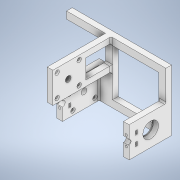
# Autodesk Inventor part: WinderBase
Saved by Autodesk Inventor 2021 (Build 250183000, 183)
## iProperties
Created: 2021-03-09
Part Number: WinderBase
Material: Generic
Document SubType Name: Modeling
Designer: elmar
Density: 1 g/cm^3
Appearance: White
Author: elmar
Autodesk Inventor part; units mm, degrees
ref_plane "YZ Plane" through (0, 0, 0) normal (1, 0, 0) x (0, 1, 0)
ref_plane "XZ Plane" through (0, 0, 0) normal (0, 1, 0) x (-1, 0, 0)
ref_plane "XY Plane" through (0, 0, 0) normal (0, 0, 1) x (1, 0, 0)
sketch "Sketch1" plane through (0, 0, 0) normal (0, 0, 1) x (1, 0, 0)
  line L0 (51, -43) -> (-51, -43)
  line L1 (-51, -43) -> (-51, 43)
  line L2 (-51, 43) -> (51, 43)
  line L3 (51, 43) -> (51, -43)
  line L4 (51, -43) -> (-51, 43) construction
  line L5 (-51, -43) -> (51, 43) construction
  point P0 (0, 0)
  dimension "d2" = 102
  dimension "d3" = 86
  constraints: 12 end point, 2 midpoint, 2 parallel, 1 horizontal, 1 perpendicular
  measures "d2" distance of L1.end L2.end
  measures "d3" distance of L0.end L1.end
extrude "Extrusion1" add sketch "Sketch1" along normal blind 8
sketch "Sketch4" plane through (0, 0, 8) normal (0, 0, 1) x (1, 0, 0)
  line L0 (-34.25, 43) -> (-26.25, 43)
  line L1 (-26.25, 43) -> (-26.25, 0)
  line L2 (-26.25, 0) -> (-34.25, 0)
  line L3 (-34.25, 0) -> (-34.25, 43)
  line L4 (51, 43) -> (-51, 43) projected
  line L5 (-51, 43) -> (-51, -43) projected
  point P0 (0, 0)
  dimension "d22" = 8
  dimension "d23" = 43
  dimension "d135" = 34.25
  constraints: 8 end point, 2 parallel, 1 collinear, 1 horizontal, 1 perpendicular
  measures "d22" distance of L0.start L0.end
  measures "d23" distance of L2.end L0.start
  measures "d135" distance from line of L3 point (0, 0)
extrude "Extrusion3" add sketch "Sketch4" along normal blind 82
sketch "Sketch5" plane through (-26.25, 0, 8) normal (1, 0, 0) x (0, 0, -1)
  circle A0 centre (-60.5, 21.5) radius 21.5
  line L0 (0, 43) -> (-82, 43) projected
  line L1 (-82, 0) -> (-82, 43) projected
  line L2 (0, 0) -> (-82, 0) projected
  line L3 (-45, 6) -> (-76, 6)
  line L4 (-76, 6) -> (-76, 37)
  line L5 (-76, 37) -> (-45, 37)
  line L6 (-45, 37) -> (-45, 6)
  line L7 (-45, 6) -> (-76, 37) construction
  line L8 (-76, 6) -> (-45, 37) construction
  point P0 (8, 0)
  dimension "d26" = 31
  constraints: 12 end point, 3 tangent, 2 midpoint, 2 parallel, 2 perpendicular, 1 centre point, 1 horizontal
  measures "d26" distance of L4.end L5.end
hole "Hole2" at (-26.25, 37, 84) at (-26.25, 37, 53) at (-26.25, 6, 53) at (-26.25, 6, 84) direction (-1, 0, 0) diameter 3.2 end through all countersink diameter 6.3 countersink angle 90 clearance for "Flat Head Machine Screw" size "M3" standard "Ansi Metric M Profile"
sketch "Sketch6" plane through (-34.25, 0, 8) normal (-1, 0, 0) x (0, 0, 1)
  point P0 (-8, 0)
  point P1 (60.5, 21.5)
hole "Hole3" at (-34.25, 21.5, 68.5) direction (1, 0, 0) diameter 8 end through all counterbore diameter 23 counterbore depth 2.2
sketch "Sketch8" plane through (0, 0, 8) normal (0, 0, 1) x (1, 0, 0)
  line L0 (51, -43) -> (51, 43) projected
  line L1 (51, -43) -> (43, -43)
  line L2 (43, -43) -> (43, 0)
  line L3 (43, 0) -> (51, 0)
  line L4 (51, 0) -> (51, -43)
  point P0 (0, 0)
  dimension "d48" = 8
  dimension "d49" = 43
  constraints: 8 end point, 2 parallel, 1 horizontal, 1 perpendicular
  measures "d48" distance of L2.end L3.end
  measures "d49" distance of L1.end L2.end
extrude "Extrusion4" add sketch "Sketch8" along normal blind 61
sketch "Sketch11" plane through (43, -43, 8) normal (-1, 0, 0) x (0, 0, 1)
  circle A0 centre (52, 21.5) radius 9
  line L0 (61, 43) -> (61, 0) projected
  point P0 (-8, 43)
  point P1 (61, 21.5)
  dimension "d67" = 18
  constraints: 1 horizontal alignment, 1 midpoint, 1 vertical, 2 other
hole "Hole7" at (43, -21.5, 60) direction (1, 0, 0) diameter 6 end through all counterbore diameter 8 counterbore depth 7
ref_plane "Work Plane1" through (46.5, -21.5, 60) normal (0, 0, 1) x (-1, 0, 0)
sketch "Sketch12" plane through (0, 0, 69) normal (0, 0, 1) x (1, 0, 0)
  line L0 (47, -17.5) -> (47, -14.5)
  line L1 (47, -25.5) -> (47, -28.5)
  line L2 (50, -17.5) -> (43, -17.5) projected
  line L3 (50, -25.5) -> (43, -25.5) projected
  line L4 (43, 0) -> (43, -43) projected
  point P0 (0, 0)
  dimension "d76" = 3
  dimension "d149" = 4
  constraints: 4 end point, 2 collinear, 2 point on line, 2 vertical
  measures "d76" distance of L0.start L0.end
  measures "d149" distance between parallel lines of L4 L0
hole "Hole8" at (47, -14.5, 69) at (47, -28.5, 69) direction (0, 0, -1) diameter 3.2 depth 30 clearance for "Flat Head Machine Screw" size "M3" standard "Ansi Metric M Profile"
sketch "Sketch16" plane through (51, -43, 0) normal (1, 0, 0) x (0, 0, -1)
  line L0 (-108, 28.5) -> (18, 28.5) projected
  line L1 (-108, 14.5) -> (18, 14.5) projected
  line L2 (-48.4, 25.75) -> (-51, 25.75)
  line L3 (-51, 25.75) -> (-51, 31.25)
  line L4 (-51, 31.25) -> (-48.4, 31.25)
  line L5 (-48.4, 31.25) -> (-48.4, 25.75)
  line L6 (-48.4, 25.75) -> (-51, 31.25) construction
  line L7 (-51, 25.75) -> (-48.4, 31.25) construction
  line L8 (-48.4, 11.75) -> (-51, 11.75)
  line L9 (-51, 11.75) -> (-51, 17.25)
  line L10 (-51, 17.25) -> (-48.4, 17.25)
  line L11 (-48.4, 17.25) -> (-48.4, 11.75)
  line L12 (-48.4, 11.75) -> (-51, 17.25) construction
  line L13 (-51, 11.75) -> (-48.4, 17.25) construction
  line L14 (-69, 0) -> (-69, 43) projected
  point P0 (0, 43)
  point P1 (-49.7, 28.5)
  point P2 (-49.7, 14.5)
  dimension "d105" = 2.6
  dimension "d106" = 5.5
  dimension "d107" = 18
  constraints: 24 end point, 4 midpoint, 4 parallel, 3 point on line, 2 collinear, 2 horizontal, 2 perpendicular
  measures "d105" distance of L3.end L4.end
  measures "d106" distance of L4.end L2.start
  measures "d107" distance between parallel lines of L14 L3
extrude "Extrusion6" cut sketch "Sketch16" against normal through all
mirror "Mirror2" about plane through (0, 0, 0) normal (1, 0, 0) of "Extrusion4", "Hole7", "Hole8", "Extrusion6"
sketch "Sketch17" plane through (-43, -43, 8) normal (1, 0, 0) x (0, 0, -1)
  circle A0 centre (-21.5, 21.5) radius 21.5
  line L0 (8, 0) -> (-61, 0) projected
  line L1 (-6, 6) -> (-37, 6)
  line L2 (-37, 6) -> (-37, 37)
  line L3 (-37, 37) -> (-6, 37)
  line L4 (-6, 37) -> (-6, 6)
  line L5 (-6, 6) -> (-37, 37) construction
  line L6 (-37, 6) -> (-6, 37) construction
  line L7 (0, 86) -> (0, 0) projected
  point P0 (8, 43)
  dimension "d110" = 31
  dimension "d139" = 43
  constraints: 12 end point, 2 midpoint, 2 parallel, 2 perpendicular, 2 tangent, 1 centre point, 1 horizontal
  measures "d110" distance of L2.end L3.end
  measures "d139" diameter of A0
hole "Hole10" at (-43, -37, 45) at (-43, -37, 14) at (-43, -6, 45) at (-43, -6, 14) direction (-1, 0, 0) diameter 3.2 depth 30 countersink diameter 6.3 countersink angle 90 clearance for "Flat Head Machine Screw" size "M3" standard "Ansi Metric M Profile"
sketch "Sketch18" plane through (-51, -43, 0) normal (-1, 0, 0) x (0, 0, 1)
  circle A0 centre (29.5, 21.5) radius 21.5 projected
  point P0 (0, 43)
hole "Hole11" at (-51, -21.5, 29.5) direction (1, 0, 0) diameter 8 end through all counterbore diameter 23 counterbore depth 2.2
split body "Split2" result two bodies by plane through (46.5, -21.5, 60) normal (0, 0, 1) first body at (-50.5, -21.5, 67) (50.5, -21.5, 67) (-26.75, 35.1569, 69.944)
sketch "Sketch19" plane through (46.5, -21.5, 60) normal (0, 0, 1) x (-1, 0, 0)
  circle A0 centre (-0.5, -7) radius 1.6 projected
  circle A1 centre (-0.5, 7) radius 1.6 projected
  line L0 (3.5, 21.5) -> (-4.5, 21.5) projected
  line L1 (-4.5, 21.5) -> (-4.5, -21.5) projected
  line L2 (-4.5, -21.5) -> (3.5, -21.5) projected
  line L3 (3.5, -21.5) -> (3.5, 21.5) projected
  circle A2 centre (93.5, -7) radius 1.6 projected
  circle A3 centre (93.5, 7) radius 1.6 projected
  line L4 (89.5, 21.5) -> (97.5, 21.5) projected
  line L5 (89.5, -21.5) -> (89.5, 21.5) projected
  line L6 (97.5, 21.5) -> (97.5, -21.5) projected
  line L7 (97.5, -21.5) -> (89.5, -21.5) projected
  point P0 (46.5, -21.5)
extrude "Extrusion7" cut sketch "Sketch19" against normal mid plane 0.4 contours L3 L2 L1 L0 | A2 | A3 | L4 L6 L7 L5 bodies 2 3
sketch "Sketch20" plane through (51, -43, 0) normal (1, 0, 0) x (0, 0, -1)
  line L0 (0, 86) -> (0, 0) projected
  line L1 (0, 0) -> (-59.8, 0) projected
  point P0 (0, 43)
  point P1 (-29.5, 21.5)
  dimension "d151" = 29.5
  dimension "d152" = 21.5
  measures "d151" distance from line of point (-29.5, 21.5) L0
  measures "d152" distance from line of point (-29.5, 21.5) L1
hole "Hole12" at (51, -21.5, 29.5) direction (-1, 0, 0) diameter 20 depth 8 counterbore diameter 22 counterbore depth 7 bodies 3
ref_plane "Work Plane2" through (-26.25, 0, 8) normal (0, -1, 0) x (0, 0, 1)
split body "Split3" result two bodies by plane through (-26.25, 0, 8) normal (0, -1, 0) bodies 2 first body at (-50.5, -21.3846, 66.9933) (50.5, -21.3846, 66.9933)
combine bodies "Combine1" operation type add bodies to combine 3 5
thicken "Thicken5" operation add thickness 10 both sides no extend neighbours yes toward (0, -1, 0) bodies 4 faces at (-48.3333, 0, 63.1333)
thicken "Thicken6" operation add thickness 10 both sides no extend neighbours yes toward (0, -1, 0) bodies 4 faces at (48.3333, 0, 63.1333)
thicken "Thicken7" operation add thickness 10 both sides no extend neighbours yes toward (0, 1, 0) bodies 4 faces at (-45.6667, -43, 63.1333)
thicken "Thicken8" operation add thickness 10 both sides no extend neighbours yes toward (0, 1, 0) bodies 4 faces at (48.3333, -43, 63.1333)
sketch "Sketch22" plane through (0, 0, 8) normal (0, 0, 1) x (1, 0, 0)
  line L0 (-26.25, 43) -> (-26.25, 0) projected
  line L1 (-43, -43) -> (43, -43) projected
  line L2 (43, -43) -> (43, 0) projected
  line L3 (43, 0) -> (51, 0) projected
  line L4 (51, 0) -> (51, 43) projected
  line L5 (51, 43) -> (-26.25, 43) projected
  line L6 (-51, 0) -> (-43, 0) projected
  line L7 (-43, 0) -> (-43, -43) projected
  line L8 (-26.25, 0) -> (-34.25, 0) projected
  line L9 (-34.25, 0) -> (-34.25, 43) projected
  line L10 (-34.25, 43) -> (-51, 43) projected
  line L11 (-51, 43) -> (-51, 0) projected
  line L12 (-24.25, -33) -> (41, -33)
  line L13 (41, -33) -> (41, 33)
  line L14 (41, 33) -> (-24.25, 33)
  line L15 (-24.25, 33) -> (-24.25, -33)
  line L16 (-34.25, 43) -> (-34.25, 0) projected
  line L17 (-51, 43) -> (-51, 0) projected
  line L18 (-34.25, 0) -> (-51, 0)
  line L19 (-51, 0) -> (-51, 43)
  line L20 (-51, 43) -> (-34.25, 43)
  line L21 (-34.25, 43) -> (-34.25, 0)
  dimension "d167" = 10
  dimension "d168" = 10
  dimension "d169" = 10
  dimension "d170" = 2
  constraints: 16 end point, 4 parallel, 2 horizontal, 2 perpendicular
  measures "d167" distance between parallel lines of L5 L14
  measures "d168" distance between parallel lines of L1 L12
  measures "d169" distance between parallel lines of L4 L13
  measures "d170" distance between parallel lines of L0 L15
extrude "Extrusion9" cut sketch "Sketch22" against normal through all contours L18 L6 L11 L10 L9 | L15 L14 L13 L12 bodies 3
sketch "Sketch23" plane through (-51, -43, 0) normal (-1, 0, 0) x (0, 0, 1)
  circle A0 centre (14, 37) radius 1.6 projected
  line L0 (0, 86) -> (90, 86) projected
  line L1 (0, 86) -> (0, 0) projected
  line L2 (8, 78) -> (43.4, 78)
  line L3 (43.4, 78) -> (43.4, 51)
  line L4 (43.4, 51) -> (8, 51)
  line L5 (8, 51) -> (8, 78)
  circle A1 centre (53, 80) radius 1.6 projected
  line L6 (8, 43) -> (90, 43) projected
  point P0 (0, 43)
  dimension "d158" = 8
  dimension "d159" = 8
  dimension "d165" = 8
  dimension "d166" = 8
  constraints: 8 end point, 2 parallel, 1 horizontal, 1 perpendicular
  measures "d158" distance between parallel lines of L1 L5
  measures "d159" distance between parallel lines of L2 L0
  measures "d165" distance between parallel lines of L6 L4
  measures "d166" distance edge to line of A1 L3
extrude "Extrusion10" cut sketch "Sketch23" against normal through all contours L2 L3 L4 L5 bodies 3
fillet "Fillet1" radius 2 8 edges at (-30.25, 8, 8) (-30.25, 35, 8) (43, -21.5, 8) (-26.25, 39, 8) (-26.25, 4, 8) (47, 0, 8) (-43, -21.5, 8) (-30.25, 0, 8)
split body "Split4" result two bodies by plane through (0, 0, 0) normal (1, 0, 0) bodies 4 first body at (50.5, -21.3846, 66.9933)
sketch "Sketch24" plane through (0, 0, 0) normal (0, 0, -1) x (-1, 0, 0)
  line L0 (-51, 43) -> (34.25, 43) projected
  line L1 (34.25, 43) -> (89, 43)
  line L2 (89, 43) -> (89, 33)
  line L3 (89, 33) -> (34.25, 33)
  line L4 (34.25, 33) -> (34.25, 43)
  line L5 (43, -43) -> (51, -43) projected
  line L6 (51, -43) -> (89, -43)
  line L7 (89, -43) -> (89, -33)
  line L8 (89, -33) -> (51, -33)
  line L9 (51, -33) -> (51, -43)
  line L10 (-41, 33) -> (24.25, 33) projected
  line L11 (24.25, -33) -> (-41, -33) projected
  line L12 (51, 0) -> (51, -43) projected
  point P0 (0, 0)
  dimension "d171" = 38
  constraints: 16 end point, 4 parallel, 3 collinear, 2 horizontal, 2 perpendicular
  measures "d171" distance between parallel lines of L12 L7
extrude "Extrusion11" add sketch "Sketch24" against normal up to surface (8 mm away) bodies 3
equation "\"dd1\" = 8"
body "Solid5"
body "Solid8"
body "Solid9"
